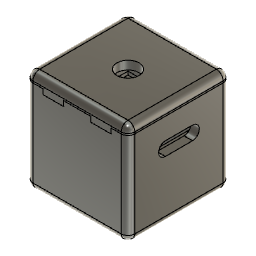
Sense board New v1 (Autodesk Fusion 360 design; units mm, degrees)
Autodesk Fusion 360 part; units mm, degrees
note: some values were not read from the file. Chosen so that the rebuilt part matches the saved one: which face or edge a step refers to. Set by a fixed rule: which sketch regions a step uses.
sketch "Sketch1" plane through (0, 0, 0) normal (0, 0, 1) x (1, 0, 0)
  line L0 (0, 0) -> (30, 0)
  line L1 (30, 0) -> (30, 30)
  line L2 (30, 30) -> (0, 30)
  line L3 (0, 30) -> (0, 0)
  dimension "d1" = 30
  dimension "d2" = 30
  constraint horizontal L0
  constraint vertical L1
  constraint horizontal L2
  constraint vertical L3
  constraint coincident L0.start L3.end
  measures "d1" distance of L0.start L0.end
  measures "d2" distance of L0.start L2.end
extrude "Extrude1" add sketch "Sketch1" along normal blind 30 makes body 1
fillet "Fillet1" radius 2 12 edges at (0, 30, 15) (0, 0, 15) (0, 15, 0) (0, 15, 30) (30, 30, 15) (15, 30, 0) (15, 30, 30) (30, 0, 15) (30, 15, 0) (30, 15, 30) (15, 0, 0) (15, 0, 30) on bodies 1
shell "Shell1" thickness 2.5 removed faces 0 bodies 1
ref_plane "WorkPlane1" through (15, 15, 27.5) normal (0, 0, 1) x (1, 0, 0)
split "Split1" by plane through (15, 15, 27.5) normal (0, 0, 1) bodies 1 makes body 2 at (10.6667, 19.3333, 30)
ref_plane "WorkPlane3" through (15, 15, 14.75) normal (0, 1, 0) x (-1, 0, 0)
ref_plane "WorkPlane4" through (15, 15, 14.75) normal (-1, 0, 0) x (0, -1, 0)
sketch "Sketch9" plane through (0, 0, 27.5) normal (0, 0, -1) x (1, 0, 0)
  arc A0 (0, -28) -> (2, -30) centre (2, -28) ccw
  line L0 (2, -30) -> (28, -30)
  arc A1 (28, -30) -> (30, -28) centre (28, -28) ccw
  line L1 (30, -28) -> (30, -2)
  arc A2 (30, -2) -> (28, 0) centre (28, -2) ccw
  line L2 (28, 0) -> (2, 0)
  arc A3 (2, 0) -> (0, -2) centre (2, -2) ccw
  line L3 (0, -2) -> (0, -28)
  line L4 (19, -19) -> (11, -19)
  line L5 (11, -19) -> (11, -11)
  line L6 (11, -11) -> (19, -11)
  line L7 (19, -11) -> (19, -19)
  line L8 (19, -19) -> (11, -11) construction
  line L9 (11, -19) -> (19, -11) construction
  line L10 (21, -21) -> (9, -21)
  line L11 (9, -21) -> (9, -9)
  line L12 (9, -9) -> (21, -9)
  line L13 (21, -9) -> (21, -21)
  line L14 (21, -21) -> (9, -9) construction
  line L15 (9, -21) -> (21, -9) construction
  point P0 (15, -15)
  point P1 (15, -15)
  dimension "d181" = 8
  dimension "d182" = 8
  dimension "d183" = 12
  dimension "d184" = 12
  constraint horizontal L4
  constraint perpendicular L4 L5
  constraint parallel L4 L6
  constraint parallel L5 L7
  constraint coincident L8 P1
  constraint coincident L9 P1
  constraint horizontal L10
  constraint perpendicular L10 L11
  constraint parallel L10 L12
  constraint parallel L11 L13
  constraint coincident L14 P1
  constraint coincident L15 P1
  constraint coincident P1 P0
  measures "d181" distance of L5.end L6.end
  measures "d182" distance of L4.end L5.end
  measures "d183" distance of L11.end L12.end
  measures "d184" distance of L10.end L11.end
sketch "Sketch8" plane through (15, 0, 0) normal (-1, 0, 0) x (0, -1, 0)
  line L0 (0, 27.5) -> (-0.9, 27.5)
  line L1 (-2, 27.5) -> (-28, 27.5)
  line L2 (0, 27.5) -> (0, 28)
  line L3 (0, 27.5) -> (0, 26)
  line L4 (0, 26) -> (-0.9, 26)
  line L5 (-1.25, 26.55) -> (-0.9, 26)
  line L6 (-1.25, 26.55) -> (-0.9, 27.1)
  line L7 (-0.9, 27.1) -> (-0.9, 27.5)
  dimension "d114" = 0.9
  dimension "d116" = 1.5
  dimension "d148" = 0.35
  dimension "d149" = 0.9
  dimension "d150" = 0.4
  constraint collinear L0 L1
  constraint coincident L0.start L2.start
  constraint perpendicular L0 L3
  constraint perpendicular L3 L4
  constraint equal L5 L6
  constraint perpendicular L0 L7
  measures "d114" distance of L3.end L4.end
  measures "d116" distance of L0.start L3.end
  measures "d148" horizontal distance of L4.end L5.start
  measures "d149" distance of L0.start L0.end
  measures "d150" distance of L0.end L6.end
extrude "Extrude10" add sketch "Sketch8" along normal blind 6 from surface at 4 bodies 2
mirror "Mirror7" about plane through (15, 15, 14.75) normal (-1, 0, 0) of "Extrude10"
mirror "Mirror8" about plane through (15, 15, 14.75) normal (0, 1, 0) of "Extrude10", "Mirror7"
combine "Combine5" operation cut target body 1 tool bodies 2 keep tools
sketch "Sketch12" plane through (25, 0, 0) normal (-1, 0, 0) x (0, -1, 0)
  line L0 (-1.25, 26.55) -> (-0.9, 26)
  line L1 (-0.9, 26) -> (0, 26)
  line L2 (0, 26) -> (0, 27.5)
  line L3 (0, 27.5) -> (-0.9, 27.5)
  line L4 (-0.9, 27.5) -> (-0.9, 27.1)
  line L5 (-0.9, 27.1) -> (-1.25, 26.55)
  line L6 (-1.1531, 27.2611) -> (-1.6056, 26.55)
  line L7 (-1.6056, 26.55) -> (-1.1531, 25.8389)
  line L8 (0, 26) -> (-1.2556, 26)
  line L9 (-1.1531, 27.2611) -> (-1.001, 27.5)
  line L10 (-1.001, 27.5) -> (0, 27.5)
  line L11 (0, 26) -> (0, 27.5)
  line L12 (-1.001, 27.5) -> (0, 27.5)
  dimension "d151" = 0.3
  constraint coincident L1.end L2.start
  constraint coincident L7 L8.end
  constraint perpendicular L2 L8
  constraint parallel L6 L9
  constraint coincident L2.end L3.start
  constraint perpendicular L2 L10
extrude "Extrude13" cut sketch "Sketch12" along normal blind 6 contours L0 L4 L5 L6 L7 L8 L9 L10 L12 bodies 1
mirror "Mirror11" about plane through (15, 15, 14.75) normal (0, 1, 0) of "Extrude13"
mirror "Mirror12" about plane through (15, 15, 14.75) normal (-1, 0, 0) of "Extrude13", "Mirror11"
sketch "Sketch13" plane through (0, 0, 30) normal (0, 0, 1) x (-1, 0, 0)
  line L0 (-2, -2) -> (-28, -2)
  line L1 (-28, -2) -> (-28, -28)
  line L2 (-28, -28) -> (-2, -28)
  line L3 (-2, -28) -> (-2, -2)
  circle A0 centre (-15, -15) radius 3.25
  dimension "d158" = 6.5
  measures "d158" diameter of A0
extrude "Extrude14" cut sketch "Sketch13" against normal blind 2.5 contours A0 bodies 2
sketch "Sketch15" plane through (2.5, 0, 0) normal (1, 0, 0) x (0, 1, 0)
  line L0 (27.5, 2.5) -> (27.5, 27.5)
  line L1 (27.5, 27.5) -> (2.5, 27.5)
  line L2 (2.5, 27.5) -> (2.5, 2.5)
  line L3 (2.5, 2.5) -> (27.5, 2.5)
  line L4 (27.5, 14.5) -> (2.5, 14.5)
  line L5 (2.5, 14.5) -> (2.5, 16)
  line L6 (2.5, 16) -> (27.5, 16)
  line L7 (27.5, 16) -> (27.5, 14.5)
  dimension "d162" = 1.5
  constraint horizontal L4
  constraint vertical L5
  constraint horizontal L6
  constraint vertical L7
  constraint coincident L0 L4.start
  measures "d162" distance of L4.start L6.end
extrude "Extrude15" add sketch "Sketch15" along normal blind 2 contours L0 L2 L4 L5 L6 L7 bodies 1
sketch "Sketch16" plane through (27.5, 0, 0) normal (-1, 0, 0) x (0, -1, 0)
  line L0 (-27.5, 27.5) -> (-27.5, 2.5)
  line L1 (-27.5, 2.5) -> (-2.5, 2.5)
  line L2 (-2.5, 2.5) -> (-2.5, 27.5)
  line L3 (-2.5, 27.5) -> (-27.5, 27.5)
  line L4 (-2.5, 14.5) -> (-27.5, 14.5)
  line L5 (-27.5, 14.5) -> (-27.5, 16)
  line L6 (-27.5, 16) -> (-2.5, 16)
  line L7 (-2.5, 16) -> (-2.5, 14.5)
  dimension "d168" = 25
  dimension "d169" = 1.5
  constraint horizontal L4
  constraint vertical L5
  constraint horizontal L6
  constraint vertical L7
  constraint coincident L2 L4.start
  measures "d168" distance of L4.start L4.end
  measures "d169" distance of L4.start L6.end
extrude "Extrude16" add sketch "Sketch16" along normal blind 2 contours L0 L2 L4 L5 L6 L7 bodies 1
sketch "Sketch17" plane through (27.5, 0, 0) normal (-1, 0, 0) x (0, -1, 0)
  line L0 (-27.5, 16) -> (-2.5, 16)
  line L1 (-2.5, 16) -> (-2.5, 27.5)
  line L2 (-2.5, 27.5) -> (-27.5, 27.5)
  line L3 (-27.5, 27.5) -> (-27.5, 16)
  line L4 (-19, 17.25) -> (-11, 17.25)
  line L5 (-20, 18.25) -> (-10, 18.25) construction
  line L6 (-19, 17.25) -> (-11, 17.25)
  arc A0 (-11, 17.25) -> (-11, 21.25) centre (-11, 19.25) ccw
  line L7 (-11, 21.25) -> (-19, 21.25)
  arc A1 (-19, 21.25) -> (-19, 17.25) centre (-19, 19.25) ccw
  line L8 (-19, 19.25) -> (-11, 19.25) construction
  dimension "d176" = 4
  constraint tangent L6 A0
  constraint tangent A0 L7
  constraint parallel L6 L7
  constraint tangent L7 A1
  constraint tangent L6 A1
  constraint parallel L5 L8
  measures "d176" diameter of A0
extrude "Extrude19" cut sketch "Sketch17" against normal blind 2.5 contours L4 L6 A0 L7 A1 bodies 1
extrude "Extrude20" add sketch "Sketch9" along normal blind 2 contours L10 L11 L12 L13 bodies 2
named bodies: "Enclosure", "Lid"
